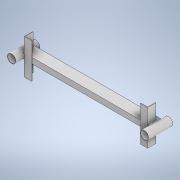
# Autodesk Inventor part: bocina2
Saved by Autodesk Inventor 2021 (Build 250183000, 183)
## iProperties
Created: 2022-01-26
Part Number: bocina2
Material: Genérico
Document SubType Name: Modeling
Designer: arthu
Density: 1 g/cm^3
Appearance: Valor por defecto
Author: arthu
Autodesk Inventor part; units mm, degrees
ref_plane "YZ Plane" through (0, 0, 0) normal (1, 0, 0) x (0, 1, 0)
ref_plane "XZ Plane" through (0, 0, 0) normal (0, 1, 0) x (-1, 0, 0)
ref_plane "XY Plane" through (0, 0, 0) normal (0, 0, 1) x (1, 0, 0)
sketch "Boceto1" plane through (0, 0, 0) normal (0, 0, 1) x (1, 0, 0)
  circle A0 centre (0, 0) radius 30
  circle A1 centre (0, 0) radius 26.15
  circle A2 centre (940, 0) radius 30
  circle A3 centre (940, 0) radius 26.15
  line L0 (22.3607, -20) -> (917.6393, -20)
  line L1 (26.15, 0) -> (30, 0)
  line L2 (910, 0) -> (940, 0)
  line L3 (22.3607, 20) -> (917.6393, 20)
  dimension "d1" = 52.3
  dimension "d0" = 60
  dimension "d2" = 940
  dimension "d3" = 60
  dimension "d4" = 52.3
  constraints: 8 end point, 6 point on circle, 4 coincident, 4 parallel, 3 centre point, 2 horizontal, 1 horizontal alignment, 2 other
  measures "d0" diameter of A0
  measures "d2" distance of point (0, 0) L2.end
  measures "d3" diameter of A2
  measures "d4" diameter of A3
extrude "Extrusión1" add sketch "Boceto1" along normal blind 80
sketch "Boceto2" plane through (0, 0, 80) normal (0, 0, 1) x (1, 0, 0)
  arc A0 (22.3607, 20) -> (22.3607, -20) centre (0, 0) ccw projected
  line L0 (22.3607, -20) -> (917.6393, -20) projected
  arc A1 (917.6393, -20) -> (917.6393, 20) centre (940, 0) ccw projected
  line L1 (917.6393, 20) -> (22.3607, 20) projected
  circle A2 centre (940, 0) radius 26.15 projected
  circle A3 centre (0, 0) radius 26.15 projected
  circle A4 centre (0, 0) radius 30
  circle A5 centre (940, 0) radius 30
  point P0 (917.6393, 20)
  point P1 (22.3607, -20)
  constraints: 2 centre point, 2 coincident
extrude "Extrusión2" add sketch "Boceto2" along normal blind 60 contours A4 A0 | A1 A5
sketch "Boceto3" plane through (0, 0, 0) normal (0, 0, -1) x (-1, 0, 0)
  arc A0 (-22.3607, -20) -> (-22.3607, 20) centre (0, 0) ccw projected
  line L0 (-917.6393, 20) -> (-22.3607, 20) projected
  arc A1 (-917.6393, 20) -> (-917.6393, -20) centre (-940, 0) ccw projected
  line L1 (-22.3607, -20) -> (-917.6393, -20) projected
  circle A2 centre (-940, 0) radius 26.15 projected
  circle A3 centre (0, 0) radius 26.15 projected
  circle A4 centre (0, 0) radius 30
  arc A5 (-917.6393, 20) -> (-917.6393, -20) centre (-940, 0) ccw projected
  circle A6 centre (-940, 0) radius 30
  point P0 (-22.3607, 20)
  constraints: 2 coincident, 6 other
extrude "Extrusión3" add sketch "Boceto3" along normal blind 30 contours A4 A0 | A1 A6
sketch "Boceto7" plane through (0, 0, 80) normal (0, 0, 1) x (1, 0, 0)
  line L0 (85, 125) -> (30, 125) projected
  line L1 (85, 20) -> (85, 125) projected
  line L2 (33.5, 125) -> (33.5, -125) projected
  line L3 (30, -125) -> (85, -125) projected
  line L4 (33.5, 125) -> (85, 125)
  line L5 (85, 125) -> (85, -125)
  line L6 (85, -125) -> (33.5, -125)
  line L7 (33.5, -125) -> (33.5, 125)
  point P0 (0, 0)
  constraints: 8 end point, 2 parallel, 1 horizontal, 1 perpendicular
extrude "Extrusión7" add sketch "Boceto7" along normal blind 3.5
sketch "Boceto8" plane through (0, 0, 80) normal (0, 0, -1) x (-1, 0, 0)
  line L0 (-33.5, -20) -> (-85, -20) projected
  line L1 (-85, -125) -> (-85, -20) projected
  line L2 (-33.5, -125) -> (-85, -125) projected
  line L3 (-33.5, -20) -> (-33.5, -125) projected
  line L4 (-85, 20) -> (-33.5, 20) projected
  line L5 (-33.5, 125) -> (-33.5, 20) projected
  line L6 (-85, 125) -> (-33.5, 125) projected
  line L7 (-85, 20) -> (-85, 125) projected
  line L8 (-33.5, 125) -> (-33.5, -125) projected
  line L9 (-85, 125) -> (-33.5, 125) projected
  line L10 (-33.5, -125) -> (-37, -125)
  line L11 (-37, -125) -> (-37, 125)
  line L12 (-37, 125) -> (-33.5, 125)
  line L13 (-33.5, 125) -> (-33.5, -125)
  line L14 (-917.6393, 20) -> (-22.3607, 20) projected
  line L15 (-470, 20) -> (-470, -237.5428)
  line L16 (-906.5, -20) -> (-855, -20)
  line L17 (-855, -125) -> (-855, -20)
  line L18 (-906.5, -125) -> (-855, -125)
  line L19 (-906.5, -20) -> (-906.5, -125)
  line L20 (-855, 20) -> (-906.5, 20)
  line L21 (-906.5, 125) -> (-906.5, 20)
  line L22 (-855, 125) -> (-906.5, 125)
  line L23 (-855, 20) -> (-855, 125)
  line L24 (-906.5, 125) -> (-906.5, -125)
  line L25 (-855, 125) -> (-906.5, 125)
  line L26 (-906.5, -125) -> (-903, -125)
  line L27 (-903, -125) -> (-903, 125)
  line L28 (-903, 125) -> (-906.5, 125)
  line L29 (-906.5, 125) -> (-906.5, -125)
  line L30 (-855, 125) -> (-903, 125)
  line L31 (-903, 125) -> (-903, -125)
  line L32 (-903, -125) -> (-855, -125)
  line L33 (-855, -125) -> (-855, 125)
  point P0 (0, 0)
  point P1 (-37, 20)
  point P2 (-37, -20)
  point P3 (-903, 20)
  point P4 (-903, -20)
  dimension "d26" = 3.5
  constraints: 46 end point, 11 symmetric about line, 4 parallel, 3 perpendicular, 2 horizontal, 2 point on line, 1 midpoint
  measures "d26" distance of L11.end L12.end
extrude "Extrusión8" add sketch "Boceto8" along normal blind 55 contours L3 L2 L11 L0 | L4 L11 L6 L5
fillet "Empalme3" radius 2 2 edges at (37, -72.5, 80) (37, 72.5, 80)
extrude "Extrusión9" add sketch "Boceto8" against normal blind 3.5 contours L33 L16 L27 L14 | L14 L27 L22 L23 | L27 L16 L24 L14 | L14 L21 L22 L27 | L17 L18 L27 L16 | L27 L18 L19 L16
extrude "Extrusión10" add sketch "Boceto8" along normal blind 55 contours L14 L21 L22 L27 | L27 L18 L19 L16
fillet "Empalme4" radius 2 2 edges at (903, -72.5, 80) (903, 72.5, 80)
